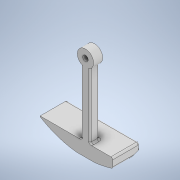
# Autodesk Inventor part: passive_walking_robot3
Saved by Autodesk Inventor 2021 (Build 250183000, 183)
## iProperties
Created: 2024-06-04
Part Number: passive_walking_robot3
Material: 一般
Document SubType Name: Modeling
Designer: 山下　響
Density: 1 g/cm^3
Appearance: 既定
Author: 山下　響
Autodesk Inventor part; units mm, degrees
ref_plane "YZ Plane" through (0, 0, 0) normal (1, 0, 0) x (0, 1, 0)
ref_plane "XZ Plane" through (0, 0, 0) normal (0, 1, 0) x (-1, 0, 0)
ref_plane "XY Plane" through (0, 0, 0) normal (0, 0, 1) x (1, 0, 0)
sketch "スケッチ1" plane through (0, 0, 0) normal (0, 0, 1) x (1, 0, 0)
  circle A0 centre (0, 0) radius 3.05
  circle A1 centre (0, 0) radius 9
  line L0 (-5, 0) -> (5, 0)
  line L1 (5, 0) -> (5, -90)
  line L2 (5, -90) -> (-5, -90)
  line L3 (-5, -90) -> (-5, 0)
  circle A2 centre (0, 0) radius 95
  line L4 (-40, -80) -> (40, -80)
  line L5 (40, -80) -> (40, -100)
  line L6 (40, -100) -> (-40, -100)
  line L7 (-40, -100) -> (-40, -80)
  line L8 (-40, -80) -> (40, -100) construction
  line L9 (40, -80) -> (-40, -100) construction
  line L10 (30, -80) -> (-50, -80)
  line L11 (-50, -80) -> (-50, -100)
  line L12 (-50, -100) -> (30, -100)
  line L13 (30, -100) -> (30, -80)
  point P0 (0, -90)
  point P1 (5, -7.4833)
  point P2 (-5, -7.4833)
  point P3 (-5, -80)
  point P4 (-40, -86.1684)
  point P5 (40, -86.1684)
  point P6 (5, -80)
  point P7 (-50, -80.7775)
  point P8 (30, -90.1388)
  dimension "d0" = 6.1
  dimension "d1" = 18
  dimension "d2" = 5
  dimension "d3" = 10
  dimension "d4" = 90
  dimension "d5" = 190
  dimension "d6" = 80
  dimension "d12" = 5
  dimension "d18" = 20
  dimension "d19" = 80
  dimension "d20" = 10
  constraints: 28 end point, 6 parallel, 3 centre point, 3 coincident, 3 horizontal, 3 midpoint, 3 perpendicular, 1 point on line
  measures "d0" diameter of A0
  measures "d1" diameter of A1
  measures "d2" distance of point (0, 0) L0.start
  measures "d3" distance of L1.end L2.end
  measures "d4" distance of L0.end L1.end
  measures "d5" diameter of A2
  measures "d6" distance of L5.end L6.end
  measures "d12" distance from line of L3 point (0, 0)
  measures "d18" distance of L6.end L4.start
  measures "d19" distance of L12.end L11.end
  measures "d20" distance between parallel lines of L5 L13
extrude "押し出し1" add sketch "スケッチ1" against normal blind 10 contours L0 L1 A1 L3 A0 | A0 L0 L3 A1 L1 | L1 L4 L3 A1
extrude "押し出し2" add sketch "スケッチ1" against normal blind 30 contours L4 L13 A2 L7 L3 L2 L1 | L1 L2 L3 L4 | L7 A2 L11 L10
sketch "スケッチ2" plane through (5, -7.4833, -10) normal (1, 0, 0) x (0, 0, -1)
  line L0 (0, 0) -> (0, 16.4833) projected
  circle A0 centre (-10, 7.4833) radius 95
  circle A1 centre (-10, 7.4833) radius 100
  circle A2 centre (20, 7.4833) radius 95
  circle A3 centre (-20, 7.4833) radius 95
  circle A4 centre (-20, 7.4833) radius 131.9121
  point P0 (5, -86.325)
  point P1 (5, 101.2916)
  point P2 (21.25, 102.4751)
  point P3 (0, 100.3542)
  point P4 (0, -85.3876)
  point P5 (-15, -87.385)
  point P6 (-63.75, -76.8431)
  dimension "d11" = 20
  dimension "d13" = 0
  dimension "d14" = 190
  dimension "d15" = 200
  dimension "d24" = 190
  dimension "d25" = 20
  dimension "d26" = 190
  constraints: 6 coincident, 5 centre point
  measures "d11" distance from line of L0 point (20, 7.483)
  measures "d13" vertical distance of point (-10, 7.483) point (20, 7.483)
  measures "d14" diameter of A0
  measures "d15" diameter of A1
  measures "d24" diameter of A2
  measures "d25" distance from line of L0 point (-20, 7.483)
  measures "d26" diameter of A3
extrude "押し出し3" cut sketch "スケッチ2" against normal mid plane 100 contours A0 A2 A3 | A0 A2 A1 | A2 A1 A3 A0 | A0 A3 A2 picked at (81.3514, 3.0261) picked at (-19.5872, -88.9746) picked at (-2.1995, -86.2848)
fillet "フィレット1" radius 2 7 edges at (30, -90.1388, -10) (-5, -43.7417, 0) (5, -43.7417, 0) (5, -43.7417, -10) (-5, -43.7417, -10) (30, -80, -15) (-50, -80.7775, -15)
fillet "フィレット2" radius 2 3 edges at (29.4142, -80.5858, -30) (30, -84.0842, -30) (-11, -80, -30)
fillet "フィレット3" radius 2 7 edges at (-4.4142, -80, -9.4142) (0, -80, -10) (4.4142, -80, -9.4142) (5, -80, -5) (4.4142, -80, -0.5858) (-4.4142, -80, -0.5858) (-5, -80, -5)
equation "\"d12\" = 0.5 * d3"
